Autodesk Inventor part; units mm, degrees
(part 3 of 4)
  line L1957 (8.8556, -3.4816) -> (8.8777, -3.4972)
  line L1958 (8.8777, -3.4972) -> (8.9019, -3.5124)
  line L1959 (8.9019, -3.5124) -> (8.9282, -3.5273)
  line L1960 (8.9282, -3.5273) -> (8.9566, -3.5418)
  line L1961 (8.9566, -3.5418) -> (8.9871, -3.5559)
  line L1962 (9.0196, -3.5695) -> (9.0542, -3.5828)
  line L1963 (11, -4.291) -> (11, -4.7124)
  line L1964 (8.7595, -3.3664) -> (8.7669, -3.3833)
  line L1965 (8.7669, -3.3833) -> (8.7764, -3.4002)
  line L1966 (8.7764, -3.4002) -> (8.788, -3.4169)
  line L1967 (8.788, -3.4169) -> (8.8018, -3.4334)
  line L1968 (8.8176, -3.4497) -> (8.8355, -3.4658)
  line L1969 (8.8355, -3.4658) -> (8.8556, -3.4816)
  line L1970 (8.8018, -3.4334) -> (8.8176, -3.4497)
  line L1971 (11, -10.5741) -> (11, -10.9956)
  line L1972 (9.0542, -9.8659) -> (11, -10.5741)
  line L1973 (9.0196, -9.8527) -> (9.0542, -9.8659)
  line L1974 (8.9871, -9.8391) -> (9.0196, -9.8527)
  line L1975 (8.788, -9.7001) -> (8.8018, -9.7166)
  line L1976 (8.8018, -9.7166) -> (8.8176, -9.7329)
  line L1977 (8.8176, -9.7329) -> (8.8355, -9.749)
  line L1978 (8.8355, -9.749) -> (8.8556, -9.7648)
  line L1979 (8.8556, -9.7648) -> (8.8777, -9.7804)
  line L1980 (8.8777, -9.7804) -> (8.9019, -9.7956)
  line L1981 (8.9019, -9.7956) -> (8.9282, -9.8105)
  line L1982 (8.9282, -9.8105) -> (8.9566, -9.825)
  line L1983 (8.9566, -9.825) -> (8.9871, -9.8391)
  line L1984 (8.7764, -9.6834) -> (8.788, -9.7001)
  line L1985 (8.7669, -9.6665) -> (8.7764, -9.6834)
  line L1986 (8.7595, -9.6495) -> (8.7669, -9.6665)
  line L1987 (8.7542, -9.6325) -> (8.7595, -9.6495)
  line L1988 (8.7511, -9.6154) -> (8.7542, -9.6325)
  line L1989 (8.75, -9.5983) -> (8.7511, -9.6154)
  line L1990 (8.75, -9.4248) -> (8.75, -9.5983)
  line L1991 (8.75, -9.4248) -> (8.75, -9.2513)
  line L1992 (8.75, -9.2513) -> (8.7511, -9.2342)
  line L1993 (8.7511, -9.2342) -> (8.7542, -9.2171)
  line L1994 (8.7542, -9.2171) -> (8.7595, -9.2)
  line L1995 (8.7595, -9.2) -> (8.7669, -9.183)
  line L1996 (8.7669, -9.183) -> (8.7764, -9.1662)
  line L1997 (8.7764, -9.1662) -> (8.788, -9.1495)
  line L1998 (8.8018, -9.133) -> (8.8176, -9.1167)
  line L1999 (8.8176, -9.1167) -> (8.8355, -9.1006)
  line L2000 (8.8355, -9.1006) -> (8.8556, -9.0847)
  line L2001 (8.8556, -9.0847) -> (8.8777, -9.0692)
  line L2002 (8.788, -9.1495) -> (8.8018, -9.133)
  line L2003 (8.8777, -9.0692) -> (8.9019, -9.054)
  line L2004 (8.9019, -9.054) -> (8.9282, -9.0391)
  line L2005 (8.9282, -9.0391) -> (8.9566, -9.0246)
  line L2006 (8.9566, -9.0246) -> (8.9871, -9.0105)
  line L2007 (8.9871, -9.0105) -> (9.0196, -8.9968)
  line L2008 (9.0196, -8.9968) -> (9.0542, -8.9836)
  line L2009 (8.8018, -6.575) -> (8.8176, -6.5913)
  line L2010 (8.8176, -6.5913) -> (8.8355, -6.6074)
  line L2011 (8.8355, -6.6074) -> (8.8556, -6.6232)
  line L2012 (8.8556, -6.6232) -> (8.8777, -6.6388)
  line L2013 (8.8777, -6.6388) -> (8.9019, -6.654)
  line L2014 (8.9019, -6.654) -> (8.9282, -6.6689)
  line L2015 (8.9282, -6.6689) -> (8.9566, -6.6834)
  line L2016 (8.9566, -6.6834) -> (8.9871, -6.6975)
  line L2017 (8.9871, -6.6975) -> (9.0196, -6.7111)
  line L2018 (8.75, 0) -> (8.75, -0.1735)
  line L2019 (8.75, -0.1735) -> (8.7511, -0.1906)
  line L2020 (8.7511, -0.1906) -> (8.7542, -0.2077)
  line L2021 (8.7542, -0.2077) -> (8.7595, -0.2248)
  line L2022 (8.7595, -0.2248) -> (8.7669, -0.2417)
  line L2023 (8.7669, -0.2417) -> (8.7764, -0.2586)
  line L2024 (8.7764, -0.2586) -> (8.788, -0.2753)
  line L2025 (8.788, -0.2753) -> (8.8018, -0.2918)
  line L2026 (9.0542, -0.4412) -> (11, -1.1494)
  line L2027 (11, -1.1494) -> (11, -1.5708)
  line L2028 (8.9566, -2.7414) -> (8.9871, -2.7273)
  line L2029 (8.9871, -2.7273) -> (9.0196, -2.7136)
  line L2030 (9.0196, -2.7136) -> (9.0542, -2.7004)
  line L2031 (11, -1.9922) -> (11, -1.5708)
  line L2032 (9.0542, -2.7004) -> (11, -1.9922)
  line L2033 (9.0542, -8.9836) -> (11, -8.2754)
  line L2034 (9.0196, -6.7111) -> (9.0542, -6.7243)
  line L2035 (9.0542, -6.7243) -> (11, -7.4326)
  line L2036 (11, -8.2754) -> (11, -7.854)
  line L2037 (11, -7.4326) -> (11, -7.854)
  line L2038 (8.7511, -34.7481) -> (8.7542, -34.7652)
  line L2039 (8.8018, -34.8493) -> (8.8176, -34.8656)
  line L2040 (8.788, -34.8328) -> (8.8018, -34.8493)
  line L2041 (8.7764, -34.8161) -> (8.788, -34.8328)
  line L2042 (8.7669, -34.7992) -> (8.7764, -34.8161)
  line L2043 (8.7595, -34.7823) -> (8.7669, -34.7992)
  line L2044 (8.75, -34.731) -> (8.7511, -34.7481)
  line L2045 (8.75, -34.5575) -> (8.75, -34.731)
  line L2046 (8.7542, -34.7652) -> (8.7595, -34.7823)
  line L2047 (8.75, -34.5575) -> (8.75, -34.384)
  line L2048 (8.75, -34.384) -> (8.7511, -34.3669)
  line L2049 (8.8556, -34.2175) -> (8.8777, -34.2019)
  line L2050 (8.8355, -34.2333) -> (8.8556, -34.2175)
  line L2051 (8.8176, -34.2494) -> (8.8355, -34.2333)
  line L2052 (8.8018, -34.2657) -> (8.8176, -34.2494)
  line L2053 (8.788, -34.2822) -> (8.8018, -34.2657)
  line L2054 (8.7764, -34.2989) -> (8.788, -34.2822)
  line L2055 (8.7669, -34.3158) -> (8.7764, -34.2989)
  line L2056 (8.7595, -34.3327) -> (8.7669, -34.3158)
  line L2057 (8.7542, -34.3498) -> (8.7595, -34.3327)
  line L2058 (8.7511, -34.3669) -> (8.7542, -34.3498)
  line L2059 (9.0542, -34.1164) -> (11, -33.4082)
  line L2060 (8.8777, -31.7715) -> (8.9019, -31.7867)
  line L2061 (8.9019, -31.7867) -> (8.9282, -31.8016)
  line L2062 (8.9282, -31.8016) -> (8.9566, -31.8161)
  line L2063 (8.9566, -31.8161) -> (8.9871, -31.8302)
  line L2064 (8.9871, -31.8302) -> (9.0196, -31.8439)
  line L2065 (9.0196, -31.8439) -> (9.0542, -31.8571)
  line L2066 (9.0542, -31.8571) -> (11, -32.5653)
  line L2067 (11, -33.4082) -> (11, -32.9867)
  line L2068 (11, -32.5653) -> (11, -32.9867)
  line L2069 (8.8176, -34.8656) -> (8.8355, -34.8817)
  line L2070 (8.8355, -34.8817) -> (8.8556, -34.8976)
  line L2071 (8.8556, -34.8976) -> (8.8777, -34.9131)
  line L2072 (8.8777, -34.9131) -> (8.9019, -34.9283)
  line L2073 (8.9019, -34.9283) -> (8.9282, -34.9432)
  line L2074 (8.9282, -34.9432) -> (8.9566, -34.9577)
  line L2075 (8.9566, -34.9577) -> (8.9871, -34.9718)
  line L2076 (8.9871, -34.9718) -> (9.0196, -34.9855)
  line L2077 (9.0196, -34.9855) -> (9.0542, -34.9987)
  line L2078 (8.8777, -34.2019) -> (8.9019, -34.1867)
  line L2079 (8.9019, -34.1867) -> (8.9282, -34.1718)
  line L2080 (8.9282, -34.1718) -> (8.9566, -34.1573)
  line L2081 (8.9566, -34.1573) -> (8.9871, -34.1432)
  line L2082 (9.0196, -34.1296) -> (9.0542, -34.1164)
  line L2083 (8.9871, -34.1432) -> (9.0196, -34.1296)
  line L2084 (8.9282, -28.66) -> (8.9566, -28.6745)
  line L2085 (8.9566, -28.6745) -> (8.9871, -28.6886)
  line L2086 (8.9871, -28.6886) -> (9.0196, -28.7023)
  line L2087 (9.0542, -28.7155) -> (11, -29.4237)
  line L2088 (8.9282, -31.0302) -> (8.9566, -31.0157)
  line L2089 (8.9566, -31.0157) -> (8.9871, -31.0016)
  line L2090 (8.9871, -31.0016) -> (9.0196, -30.988)
  line L2091 (9.0542, -30.9748) -> (11, -30.2666)
  line L2092 (11, -30.2666) -> (11, -29.8451)
  line L2093 (11, -29.4237) -> (11, -29.8451)
  line L2094 (9.0196, -28.7023) -> (9.0542, -28.7155)
  line L2095 (9.0196, -30.988) -> (9.0542, -30.9748)
  line L2096 (8.75, -6.2832) -> (7.8414, -6.2832)
  line L2097 (8.75, -6.2832) -> (8.75, -6.4567)
  line L2098 (8.75, -6.4567) -> (8.7511, -6.4738)
  line L2099 (8.7511, -6.4738) -> (8.7542, -6.4909)
  line L2100 (8.7542, -6.4909) -> (8.7595, -6.508)
  line L2101 (8.7595, -6.508) -> (8.7669, -6.5249)
  line L2102 (8.7669, -6.5249) -> (8.7764, -6.5418)
  line L2103 (8.7764, -6.5418) -> (8.788, -6.5585)
  line L2104 (8.788, -6.5585) -> (8.8018, -6.575)
  line L2105 (9.0542, -34.9987) -> (11, -35.7069)
  line L2106 (11, -35.7069) -> (11, -36.1283)
  line L2107 (11, -36.5497) -> (11, -36.1283)
  line L2108 (9.0542, -37.258) -> (11, -36.5497)
  line L2109 (9.0196, -37.2712) -> (9.0542, -37.258)
  line L2110 (8.9871, -37.2848) -> (9.0196, -37.2712)
  line L2111 (8.9566, -37.2989) -> (8.9871, -37.2848)
  line L2112 (8.9282, -37.3134) -> (8.9566, -37.2989)
  line L2113 (8.9019, -37.3283) -> (8.9282, -37.3134)
  line L2114 (8.8777, -37.3435) -> (8.9019, -37.3283)
  line L2115 (8.8556, -37.3591) -> (8.8777, -37.3435)
  line L2116 (8.788, -75.123) -> (8.8018, -75.1064)
  line L2117 (8.7764, -75.1397) -> (8.788, -75.123)
  line L2118 (8.7669, -75.1565) -> (8.7764, -75.1397)
  line L2119 (8.7595, -75.1735) -> (8.7669, -75.1565)
  line L2120 (8.7542, -75.1905) -> (8.7595, -75.1735)
  line L2121 (8.7511, -75.2076) -> (8.7542, -75.1905)
  line L2122 (8.75, -75.2247) -> (8.7511, -75.2076)
  line L2123 (8.75, -75.3982) -> (8.75, -75.2247)
  line L2124 (9.0196, -72.6846) -> (9.0542, -72.6978)
  line L2125 (8.9871, -72.6709) -> (9.0196, -72.6846)
  line L2126 (8.9566, -72.6568) -> (8.9871, -72.6709)
  line L2127 (8.9282, -72.6423) -> (8.9566, -72.6568)
  line L2128 (8.9019, -72.6274) -> (8.9282, -72.6423)
  line L2129 (8.8777, -72.6122) -> (8.9019, -72.6274)
  line L2130 (8.8556, -72.5967) -> (8.8777, -72.6122)
  line L2131 (8.8355, -72.5808) -> (8.8556, -72.5967)
  line L2132 (8.8176, -72.5648) -> (8.8355, -72.5808)
  line L2133 (8.8018, -72.5484) -> (8.8176, -72.5648)
  line L2134 (8.788, -72.5319) -> (8.8018, -72.5484)
  line L2135 (8.7764, -72.5152) -> (8.788, -72.5319)
  line L2136 (8.8176, -75.0901) -> (8.8355, -75.074)
  line L2137 (8.8018, -75.1064) -> (8.8176, -75.0901)
  line L2138 (8.8355, -75.074) -> (8.8556, -75.0582)
  line L2139 (8.8556, -75.0582) -> (8.8777, -75.0426)
  line L2140 (8.8777, -75.0426) -> (8.9019, -75.0274)
  line L2141 (8.9019, -75.0274) -> (8.9282, -75.0125)
  line L2142 (8.9282, -75.0125) -> (8.9566, -74.998)
  line L2143 (8.9566, -74.998) -> (8.9871, -74.9839)
  line L2144 (8.9871, -74.9839) -> (9.0196, -74.9703)
  line L2145 (8.7669, -72.4984) -> (8.7764, -72.5152)
  line L2146 (8.7595, -72.4814) -> (8.7669, -72.4984)
  line L2147 (8.7542, -72.4644) -> (8.7595, -72.4814)
  line L2148 (8.7511, -72.4472) -> (8.7542, -72.4644)
  line L2149 (8.75, -72.4301) -> (8.7511, -72.4472)
  line L2150 (8.75, -72.2566) -> (8.75, -72.4301)
  line L2151 (8.75, -72.2566) -> (8.75, -72.0831)
  line L2152 (8.75, -72.0831) -> (8.7511, -72.066)
  line L2153 (8.7511, -72.066) -> (8.7542, -72.0489)
  line L2154 (8.7542, -72.0489) -> (8.7595, -72.0319)
  line L2155 (8.7595, -72.0319) -> (8.7669, -72.0149)
  line L2156 (8.7669, -72.0149) -> (8.7764, -71.9981)
  line L2157 (8.7595, -69.3398) -> (8.7669, -69.3568)
  line L2158 (8.7542, -69.3228) -> (8.7595, -69.3398)
  line L2159 (8.7511, -69.3057) -> (8.7542, -69.3228)
  line L2160 (8.75, -69.2885) -> (8.7511, -69.3057)
  line L2161 (8.75, -69.115) -> (8.75, -69.2885)
  line L2162 (8.7764, -71.9981) -> (8.788, -71.9814)
  line L2163 (8.788, -71.9814) -> (8.8018, -71.9648)
  line L2164 (8.8018, -71.9648) -> (8.8176, -71.9485)
  line L2165 (8.8176, -71.9485) -> (8.8355, -71.9324)
  line L2166 (8.8355, -71.9324) -> (8.8556, -71.9166)
  line L2167 (8.8556, -71.9166) -> (8.8777, -71.901)
  line L2168 (8.8777, -71.901) -> (8.9019, -71.8858)
  line L2169 (8.9019, -71.8858) -> (8.9282, -71.8709)
  line L2170 (8.7669, -69.3568) -> (8.7764, -69.3736)
  line L2171 (8.9871, -71.8423) -> (9.0196, -71.8287)
  line L2172 (8.9566, -71.8564) -> (8.9871, -71.8423)
  line L2173 (8.9282, -71.8709) -> (8.9566, -71.8564)
  line L2174 (9.0542, -69.5562) -> (11, -70.2644)
  line L2175 (9.0196, -71.8287) -> (9.0542, -71.8155)
  line L2176 (9.0542, -71.8155) -> (11, -71.1073)
  line L2177 (11, -70.2644) -> (11, -70.6858)
  line L2178 (11, -71.1073) -> (11, -70.6858)
  line L2179 (8.7764, -68.8565) -> (8.788, -68.8398)
  line L2180 (8.788, -68.8398) -> (8.8018, -68.8232)
  line L2181 (8.8018, -68.8232) -> (8.8176, -68.8069)
  line L2182 (8.8176, -68.8069) -> (8.8355, -68.7908)
  line L2183 (8.8355, -68.7908) -> (8.8556, -68.775)
  line L2184 (8.8556, -68.775) -> (8.8777, -68.7595)
  line L2185 (9.0196, -68.6871) -> (9.0542, -68.6739)
  line L2186 (8.9871, -68.7008) -> (9.0196, -68.6871)
  line L2187 (8.9566, -68.7149) -> (8.9871, -68.7008)
  line L2188 (8.9282, -68.7294) -> (8.9566, -68.7149)
  line L2189 (8.8777, -68.7595) -> (8.9019, -68.7442)
  line L2190 (8.9019, -68.7442) -> (8.9282, -68.7294)
  line L2191 (9.0542, -68.6739) -> (11, -67.9657)
  line L2192 (11, -67.9657) -> (11, -67.5442)
  line L2193 (11, -67.1228) -> (11, -67.5442)
  line L2194 (9.0542, -66.4146) -> (11, -67.1228)
  line L2195 (9.0196, -66.4014) -> (9.0542, -66.4146)
  line L2196 (8.9871, -66.3877) -> (9.0196, -66.4014)
  line L2197 (8.9566, -66.3736) -> (8.9871, -66.3877)
  line L2198 (8.9282, -66.3591) -> (8.9566, -66.3736)
  line L2199 (8.9019, -66.3443) -> (8.9282, -66.3591)
  line L2200 (8.8777, -66.329) -> (8.9019, -66.3443)
  line L2201 (8.8556, -66.3135) -> (8.8777, -66.329)
  line L2202 (8.8355, -66.2977) -> (8.8556, -66.3135)
  line L2203 (8.8176, -66.2816) -> (8.8355, -66.2977)
  line L2204 (8.8018, -66.2652) -> (8.8176, -66.2816)
  line L2205 (8.788, -66.2487) -> (8.8018, -66.2652)
  line L2206 (8.7764, -66.232) -> (8.788, -66.2487)
  line L2207 (8.7669, -66.2152) -> (8.7764, -66.232)
  line L2208 (8.7595, -66.1982) -> (8.7669, -66.2152)
  line L2209 (8.7511, -66.1641) -> (8.7542, -66.1812)
  line L2210 (8.7542, -66.1812) -> (8.7595, -66.1982)
  line L2211 (8.75, -65.9734) -> (8.75, -65.8)
  line L2212 (8.75, -65.8) -> (8.7511, -65.7828)
  line L2213 (8.7511, -65.7828) -> (8.7542, -65.7657)
  line L2214 (8.7542, -65.7657) -> (8.7595, -65.7487)
  line L2215 (8.7595, -65.7487) -> (8.7669, -65.7317)
  line L2216 (8.7669, -65.7317) -> (8.7764, -65.7149)
  line L2217 (8.7764, -65.7149) -> (8.788, -65.6982)
  line L2218 (8.788, -65.6982) -> (8.8018, -65.6816)
  line L2219 (8.8018, -65.6816) -> (8.8176, -65.6653)
  line L2220 (8.8176, -65.6653) -> (8.8355, -65.6492)
  line L2221 (8.8355, -65.6492) -> (8.8556, -65.6334)
  line L2222 (8.8556, -65.6334) -> (8.8777, -65.6179)
  line L2223 (8.8777, -65.6179) -> (8.9019, -65.6026)
  line L2224 (8.9019, -65.6026) -> (8.9282, -65.5878)
  line L2225 (8.9566, -65.5733) -> (8.9871, -65.5592)
  line L2226 (8.9871, -65.5592) -> (9.0196, -65.5455)
  line L2227 (9.0196, -65.5455) -> (9.0542, -65.5323)
  line L2228 (8.9282, -65.5878) -> (8.9566, -65.5733)
  line L2229 (11, -64.8241) -> (11, -64.4026)
  line L2230 (9.0542, -63.273) -> (11, -63.9812)
  line L2231 (9.0542, -65.5323) -> (11, -64.8241)
  line L2232 (11, -63.9812) -> (11, -64.4026)
  line L2233 (9.0196, -69.543) -> (9.0542, -69.5562)
  line L2234 (8.9871, -69.5293) -> (9.0196, -69.543)
  line L2235 (8.9566, -69.5152) -> (8.9871, -69.5293)
  line L2236 (8.9282, -69.5007) -> (8.9566, -69.5152)
  line L2237 (8.9019, -69.4858) -> (8.9282, -69.5007)
  line L2238 (8.8556, -69.4551) -> (8.8777, -69.4706)
  line L2239 (8.8355, -69.4392) -> (8.8556, -69.4551)
  line L2240 (8.8176, -69.4232) -> (8.8355, -69.4392)
  line L2241 (8.8018, -69.4068) -> (8.8176, -69.4232)
  line L2242 (8.788, -69.3903) -> (8.8018, -69.4068)
  line L2243 (8.7764, -69.3736) -> (8.788, -69.3903)
  line L2244 (8.8777, -69.4706) -> (8.9019, -69.4858)
  line L2245 (9.0542, -72.6978) -> (11, -73.406)
  line L2246 (11, -73.406) -> (11, -73.8274)
  line L2247 (11, -74.2489) -> (11, -73.8274)
  line L2248 (9.0542, -74.9571) -> (11, -74.2489)
  line L2249 (9.0196, -74.9703) -> (9.0542, -74.9571)
  line L2250 (8.75, -75.3982) -> (8.75, -75.5717)
  line L2251 (8.75, -75.5717) -> (8.7511, -75.5888)
  line L2252 (8.7511, -75.5888) -> (8.7542, -75.6059)
  line L2253 (8.7542, -75.6059) -> (8.7595, -75.623)
  line L2254 (8.7595, -75.623) -> (8.7669, -75.64)
  line L2255 (8.7669, -75.64) -> (8.7764, -75.6568)
  line L2256 (8.7764, -75.6568) -> (8.788, -75.6735)
  line L2257 (8.788, -75.6735) -> (8.8018, -75.69)
  line L2258 (8.8176, -75.7063) -> (8.8355, -75.7224)
  line L2259 (8.8018, -75.69) -> (8.8176, -75.7063)
  line L2260 (8.8355, -75.7224) -> (8.8556, -75.7383)
  line L2261 (8.8777, -75.7538) -> (8.9019, -75.769)
  line L2262 (8.9019, -75.769) -> (8.9282, -75.7839)
  line L2263 (8.9282, -75.7839) -> (8.9566, -75.7984)
  line L2264 (8.9566, -75.7984) -> (8.9871, -75.8125)
  line L2265 (8.8556, -75.7383) -> (8.8777, -75.7538)
  line L2266 (9.0196, -63.2598) -> (9.0542, -63.273)
  line L2267 (8.9871, -63.2461) -> (9.0196, -63.2598)
  line L2268 (8.9566, -63.232) -> (8.9871, -63.2461)
  line L2269 (8.9282, -63.2175) -> (8.9566, -63.232)
  line L2270 (8.9019, -63.2027) -> (8.9282, -63.2175)
  line L2271 (8.8777, -63.1874) -> (8.9019, -63.2027)
  line L2272 (8.8556, -63.1719) -> (8.8777, -63.1874)
  line L2273 (8.8355, -63.1561) -> (8.8556, -63.1719)
  line L2274 (8.7669, -63.0736) -> (8.7764, -63.0904)
  line L2275 (8.7595, -63.0566) -> (8.7669, -63.0736)
  line L2276 (8.7542, -63.0396) -> (8.7595, -63.0566)
  line L2277 (8.7511, -63.0225) -> (8.7542, -63.0396)
  line L2278 (8.75, -63.0053) -> (8.7511, -63.0225)
  line L2279 (8.75, -62.8319) -> (8.75, -63.0053)
  line L2280 (9.0196, -88.3925) -> (9.0542, -88.4058)
  line L2281 (9.0542, -88.4058) -> (11, -89.114)
  line L2282 (8.9566, -90.706) -> (8.9871, -90.6919)
  line L2283 (8.9871, -90.6919) -> (9.0196, -90.6782)
  line L2284 (9.0196, -90.6782) -> (9.0542, -90.665)
  line L2285 (9.0542, -90.665) -> (11, -89.9568)
  line L2286 (11, -89.9568) -> (11, -89.5354)
  line L2287 (11, -89.114) -> (11, -89.5354)
  line L2288 (8.9282, -90.7205) -> (8.9566, -90.706)
  line L2289 (8.7669, -90.8645) -> (8.7764, -90.8476)
  line L2290 (8.9019, -90.7354) -> (8.9282, -90.7205)
  line L2291 (8.8777, -90.7506) -> (8.9019, -90.7354)
  line L2292 (8.8556, -90.7661) -> (8.8777, -90.7506)
  line L2293 (8.8355, -90.782) -> (8.8556, -90.7661)
  line L2294 (8.8176, -90.7981) -> (8.8355, -90.782)
  line L2295 (8.8018, -90.8144) -> (8.8176, -90.7981)
  line L2296 (8.788, -90.8309) -> (8.8018, -90.8144)
  line L2297 (8.75, -91.1062) -> (8.75, -90.9327)
  line L2298 (8.75, -91.1062) -> (8.75, -91.2797)
  line L2299 (8.7764, -90.8476) -> (8.788, -90.8309)
  line L2300 (8.75, -91.2797) -> (8.7511, -91.2968)
  line L2301 (8.7511, -91.2968) -> (8.7542, -91.3139)
  line L2302 (8.7542, -91.3139) -> (8.7595, -91.331)
  line L2303 (8.7595, -91.331) -> (8.7669, -91.3479)
  line L2304 (8.7669, -91.3479) -> (8.7764, -91.3648)
  line L2305 (8.7764, -91.3648) -> (8.788, -91.3815)
  line L2306 (8.788, -91.3815) -> (8.8018, -91.398)
  line L2307 (8.8018, -91.398) -> (8.8176, -91.4143)
  line L2308 (8.8176, -91.4143) -> (8.8355, -91.4304)
  line L2309 (8.8355, -91.4304) -> (8.8556, -91.4462)
  line L2310 (8.8556, -91.4462) -> (8.8777, -91.4618)
  line L2311 (8.8777, -91.4618) -> (8.9019, -91.477)
  line L2312 (8.9019, -91.477) -> (8.9282, -91.4919)
  line L2313 (8.9282, -91.4919) -> (8.9566, -91.5064)
  line L2314 (8.9566, -91.5064) -> (8.9871, -91.5205)
  line L2315 (8.9871, -91.5205) -> (9.0196, -91.5341)
  line L2316 (9.0196, -91.5341) -> (9.0542, -91.5473)
  line L2317 (8.9871, -93.8335) -> (9.0196, -93.8198)
  line L2318 (9.0196, -93.8198) -> (9.0542, -93.8066)
  line L2319 (9.0542, -93.8066) -> (11, -93.0984)
  line L2320 (11, -93.0984) -> (11, -92.677)
  line L2321 (11, -92.2556) -> (11, -92.677)
  line L2322 (9.0542, -91.5473) -> (11, -92.2556)
  line L2323 (8.9566, -93.8476) -> (8.9871, -93.8335)
  line L2324 (8.75, -90.9327) -> (8.7511, -90.9156)
  line L2325 (8.7669, -94.0061) -> (8.7764, -93.9892)
  line L2326 (8.7511, -94.0572) -> (8.7542, -94.0401)
  line L2327 (8.75, -94.0743) -> (8.7511, -94.0572)
  line L2328 (8.75, -94.2478) -> (7.8414, -94.2478)
  line L2329 (8.75, -94.2478) -> (8.75, -94.0743)
  line L2330 (8.7595, -94.023) -> (8.7669, -94.0061)
  line L2331 (8.9282, -93.8621) -> (8.9566, -93.8476)
  line L2332 (8.9019, -93.877) -> (8.9282, -93.8621)
  line L2333 (8.8777, -93.8922) -> (8.9019, -93.877)
  line L2334 (8.8556, -93.9077) -> (8.8777, -93.8922)
  line L2335 (8.8355, -93.9236) -> (8.8556, -93.9077)
  line L2336 (8.8176, -93.9397) -> (8.8355, -93.9236)
  line L2337 (8.8018, -93.956) -> (8.8176, -93.9397)
  line L2338 (8.788, -93.9725) -> (8.8018, -93.956)
  line L2339 (8.7764, -93.9892) -> (8.788, -93.9725)
  line L2340 (8.7542, -94.0401) -> (8.7595, -94.023)
  line L2341 (8.75, -94.2478) -> (8.75, -94.4213)
  line L2342 (8.75, -94.4213) -> (8.7511, -94.4384)
  line L2343 (8.7511, -94.4384) -> (8.7542, -94.4555)
  line L2344 (8.7595, -94.4725) -> (8.7669, -94.4895)
  line L2345 (8.7669, -94.4895) -> (8.7764, -94.5064)
  line L2346 (8.7542, -94.4555) -> (8.7595, -94.4725)
  line L2347 (8.9282, -97.0037) -> (8.9566, -96.9892)
  line L2348 (8.9019, -97.0186) -> (8.9282, -97.0037)
  line L2349 (8.8777, -97.0338) -> (8.9019, -97.0186)
  line L2350 (8.8556, -97.0493) -> (8.8777, -97.0338)
  line L2351 (8.8176, -97.0813) -> (8.8355, -97.0652)
  line L2352 (8.8018, -97.0976) -> (8.8176, -97.0813)
  line L2353 (8.788, -97.1141) -> (8.8018, -97.0976)
  line L2354 (8.7764, -97.1308) -> (8.788, -97.1141)
  line L2355 (8.7595, -97.1646) -> (8.7669, -97.1476)
  line L2356 (8.7542, -97.1816) -> (8.7595, -97.1646)
  line L2357 (8.7511, -97.1988) -> (8.7542, -97.1816)
  line L2358 (8.8355, -97.0652) -> (8.8556, -97.0493)
  line L2359 (8.75, -97.3894) -> (8.75, -97.2159)
  line L2360 (8.75, -97.3894) -> (8.75, -97.5629)
  line L2361 (8.75, -97.5629) -> (8.7511, -97.58)
  line L2362 (8.7511, -97.58) -> (8.7542, -97.5971)
  line L2363 (8.7542, -97.5971) -> (8.7595, -97.6141)
  line L2364 (8.7595, -97.6141) -> (8.7669, -97.6311)
  line L2365 (8.75, -97.2159) -> (8.7511, -97.1988)
  line L2366 (8.8777, -94.6034) -> (8.9019, -94.6186)
  line L2367 (8.9019, -94.6186) -> (8.9282, -94.6335)
  line L2368 (8.9282, -94.6335) -> (8.9566, -94.648)
  line L2369 (8.8556, -94.5878) -> (8.8777, -94.6034)
  line L2370 (8.7764, -94.5064) -> (8.788, -94.5231)
  line L2371 (8.788, -94.5231) -> (8.8018, -94.5396)
  line L2372 (8.8018, -94.5396) -> (8.8176, -94.5559)
  line L2373 (8.8176, -94.5559) -> (8.8355, -94.572)
  line L2374 (8.8355, -94.572) -> (8.8556, -94.5878)
  line L2375 (8.7669, -97.1476) -> (8.7764, -97.1308)
  line L2376 (8.7669, -97.6311) -> (8.7764, -97.6479)
  line L2377 (8.788, -97.6646) -> (8.8018, -97.6812)
  line L2378 (8.8018, -97.6812) -> (8.8176, -97.6975)
  line L2379 (8.8176, -97.6975) -> (8.8355, -97.7136)
  line L2380 (8.8355, -97.7136) -> (8.8556, -97.7294)
  line L2381 (8.8556, -97.7294) -> (8.8777, -97.745)
  line L2382 (8.7764, -97.6479) -> (8.788, -97.6646)
  line L2383 (8.8777, -97.745) -> (8.9019, -97.7602)
  line L2384 (8.9019, -97.7602) -> (8.9282, -97.7751)
  line L2385 (8.9566, -97.7896) -> (8.9871, -97.8037)
  line L2386 (8.9871, -97.8037) -> (9.0196, -97.8173)
  line L2387 (9.0196, -97.8173) -> (9.0542, -97.8305)
  line L2388 (9.0542, -97.8305) -> (11, -98.5387)
  line L2389 (11, -98.5387) -> (11, -98.9602)
  line L2390 (8.9282, -97.7751) -> (8.9566, -97.7896)
  line L2391 (8.9566, -94.648) -> (8.9871, -94.6621)
  line L2392 (8.9871, -94.6621) -> (9.0196, -94.6757)
  line L2393 (9.0196, -94.6757) -> (9.0542, -94.6889)
  line L2394 (9.0542, -94.6889) -> (11, -95.3971)
  line L2395 (11, -95.3971) -> (11, -95.8186)
  line L2396 (8.9871, -96.9751) -> (9.0196, -96.9614)
  line L2397 (9.0196, -96.9614) -> (9.0542, -96.9482)
  line L2398 (9.0542, -96.9482) -> (11, -96.24)
  line L2399 (11, -96.24) -> (11, -95.8186)
  line L2400 (8.9566, -96.9892) -> (8.9871, -96.9751)
  line L2401 (9.0542, -85.2642) -> (11, -85.9724)
  line L2402 (9.0542, -87.5234) -> (11, -86.8152)
  line L2403 (11, -85.9724) -> (11, -86.3938)
  line L2404 (11, -86.8152) -> (11, -86.3938)
  line L2405 (8.9871, -85.2373) -> (9.0196, -85.251)
  line L2406 (8.9871, -75.8125) -> (9.0196, -75.8262)
  line L2407 (9.0196, -75.8262) -> (9.0542, -75.8394)
  line L2408 (9.0542, -75.8394) -> (11, -76.5476)
  line L2409 (11, -76.5476) -> (11, -76.969)
  line L2410 (11, -77.3904) -> (11, -76.969)
  line L2411 (9.0542, -78.0987) -> (11, -77.3904)
  line L2412 (9.0196, -78.1119) -> (9.0542, -78.0987)
  line L2413 (8.8018, -78.248) -> (8.8176, -78.2317)
  line L2414 (8.8176, -78.2317) -> (8.8355, -78.2156)
  line L2415 (8.8355, -78.2156) -> (8.8556, -78.1998)
  line L2416 (8.8556, -78.1998) -> (8.8777, -78.1842)
  line L2417 (8.8777, -78.1842) -> (8.9019, -78.169)
  line L2418 (8.9019, -78.169) -> (8.9282, -78.1541)
  line L2419 (8.9282, -78.1541) -> (8.9566, -78.1396)
  line L2420 (8.9566, -78.1396) -> (8.9871, -78.1255)
  line L2421 (8.9871, -78.1255) -> (9.0196, -78.1119)
  line L2422 (8.7511, -78.3492) -> (8.7542, -78.3321)
  line L2423 (8.788, -78.8151) -> (8.8018, -78.8316)
  line L2424 (8.7764, -78.7984) -> (8.788, -78.8151)
  line L2425 (8.7669, -78.7815) -> (8.7764, -78.7984)
  line L2426 (8.7595, -78.7646) -> (8.7669, -78.7815)
  line L2427 (8.7542, -78.7475) -> (8.7595, -78.7646)
  line L2428 (8.7511, -78.7304) -> (8.7542, -78.7475)
  line L2429 (8.75, -78.5398) -> (8.75, -78.7133)
  line L2430 (8.75, -78.5398) -> (8.75, -78.3663)
  line L2431 (8.75, -78.3663) -> (8.7511, -78.3492)
  line L2432 (8.7542, -78.3321) -> (8.7595, -78.315)
  line L2433 (8.7595, -78.315) -> (8.7669, -78.2981)
  line L2434 (8.7669, -78.2981) -> (8.7764, -78.2812)
  line L2435 (8.7764, -78.2812) -> (8.788, -78.2645)
  line L2436 (8.788, -78.2645) -> (8.8018, -78.248)
  line L2437 (8.75, -78.7133) -> (8.7511, -78.7304)
  line L2438 (9.0196, -78.9678) -> (9.0542, -78.981)
  line L2439 (8.9871, -78.9541) -> (9.0196, -78.9678)
  line L2440 (8.9566, -78.94) -> (8.9871, -78.9541)
  line L2441 (8.9282, -78.9255) -> (8.9566, -78.94)
  line L2442 (8.9019, -78.9106) -> (8.9282, -78.9255)
  line L2443 (8.8777, -78.8954) -> (8.9019, -78.9106)
  line L2444 (8.8556, -78.8799) -> (8.8777, -78.8954)
  line L2445 (8.8355, -78.864) -> (8.8556, -78.8799)
  line L2446 (8.8176, -78.8479) -> (8.8355, -78.864)
  line L2447 (8.8018, -78.8316) -> (8.8176, -78.8479)
  line L2448 (9.0196, -81.2535) -> (9.0542, -81.2402)
  line L2449 (9.0542, -78.981) -> (11, -79.6892)
  line L2450 (8.9282, -81.2957) -> (8.9566, -81.2812)
  line L2451 (8.9566, -81.2812) -> (8.9871, -81.2671)
  line L2452 (8.9871, -81.2671) -> (9.0196, -81.2535)
  line L2453 (9.0542, -81.2402) -> (11, -80.532)
  line L2454 (11, -79.6892) -> (11, -80.1106)
  line L2455 (11, -80.532) -> (11, -80.1106)
  line L2456 (8.7542, -81.8891) -> (8.7595, -81.9062)
  line L2457 (8.7511, -81.872) -> (8.7542, -81.8891)
  line L2458 (8.75, -81.8549) -> (8.7511, -81.872)
  line L2459 (8.75, -81.6814) -> (8.75, -81.8549)
  line L2460 (8.75, -81.6814) -> (8.75, -81.5079)
  line L2461 (8.75, -81.5079) -> (8.7511, -81.4908)
  line L2462 (8.7511, -81.4908) -> (8.7542, -81.4737)
  line L2463 (8.7542, -81.4737) -> (8.7595, -81.4566)
  line L2464 (9.0542, -84.3818) -> (11, -83.6736)
  line L2465 (9.0542, -82.1226) -> (11, -82.8308)
  line L2466 (11, -82.8308) -> (11, -83.2522)
  line L2467 (11, -83.6736) -> (11, -83.2522)
  line L2468 (8.7595, -84.5982) -> (8.7669, -84.5813)
  line L2469 (8.7669, -84.5813) -> (8.7764, -84.5644)
  line L2470 (8.7764, -84.5644) -> (8.788, -84.5477)
  line L2471 (8.788, -84.5477) -> (8.8018, -84.5312)
  line L2472 (8.8018, -84.5312) -> (8.8176, -84.5149)
  line L2473 (8.8176, -84.5149) -> (8.8355, -84.4988)
  line L2474 (8.8355, -84.4988) -> (8.8556, -84.483)
  line L2475 (8.8556, -84.483) -> (8.8777, -84.4674)
  line L2476 (8.8777, -84.4674) -> (8.9019, -84.4522)
  line L2477 (8.9019, -84.4522) -> (8.9282, -84.4373)
  line L2478 (8.9282, -84.4373) -> (8.9566, -84.4228)
  line L2479 (8.9566, -84.4228) -> (8.9871, -84.4087)
  line L2480 (8.9871, -84.4087) -> (9.0196, -84.395)
  line L2481 (9.0196, -84.395) -> (9.0542, -84.3818)
  line L2482 (8.7542, -84.6153) -> (8.7595, -84.5982)
  line L2483 (8.7511, -84.6324) -> (8.7542, -84.6153)
  line L2484 (8.75, -84.6495) -> (8.7511, -84.6324)
  line L2485 (8.75, -84.823) -> (8.75, -84.6495)
  line L2486 (8.75, -84.823) -> (8.75, -84.9965)
  line L2487 (8.75, -84.9965) -> (8.7511, -85.0136)
  line L2488 (8.7511, -85.0136) -> (8.7542, -85.0307)
  line L2489 (8.7542, -85.0307) -> (8.7595, -85.0478)
  line L2490 (8.8018, -85.1148) -> (8.8176, -85.1311)
  line L2491 (8.788, -85.0983) -> (8.8018, -85.1148)
  line L2492 (8.7669, -85.0647) -> (8.7764, -85.0816)
  line L2493 (8.7764, -85.0816) -> (8.788, -85.0983)
  line L2494 (8.8176, -85.1311) -> (8.8355, -85.1472)
  line L2495 (8.7595, -85.0478) -> (8.7669, -85.0647)
  line L2496 (8.9019, -85.1938) -> (8.9282, -85.2087)
  line L2497 (8.9282, -85.2087) -> (8.9566, -85.2232)
  line L2498 (8.7669, -87.7229) -> (8.7764, -87.706)
  line L2499 (8.9566, -87.5644) -> (8.9871, -87.5503)
  line L2500 (8.9871, -87.5503) -> (9.0196, -87.5366)
  line L2501 (9.0196, -87.5366) -> (9.0542, -87.5234)
  line L2502 (8.9282, -87.5789) -> (8.9566, -87.5644)
  line L2503 (8.9019, -87.5938) -> (8.9282, -87.5789)
  line L2504 (8.8777, -87.609) -> (8.9019, -87.5938)
  line L2505 (8.8355, -87.6404) -> (8.8556, -87.6246)
  line L2506 (8.8176, -87.6565) -> (8.8355, -87.6404)
  line L2507 (8.8018, -87.6728) -> (8.8176, -87.6565)
  line L2508 (8.788, -87.6893) -> (8.8018, -87.6728)
  line L2509 (8.7764, -87.706) -> (8.788, -87.6893)
  line L2510 (8.8556, -87.6246) -> (8.8777, -87.609)
  line L2511 (8.75, -87.7911) -> (8.7511, -87.774)
  line L2512 (8.7511, -87.774) -> (8.7542, -87.7569)
  line L2513 (8.7542, -87.7569) -> (8.7595, -87.7398)
  line L2514 (8.7595, -87.7398) -> (8.7669, -87.7229)
  line L2515 (8.75, -87.9646) -> (8.75, -87.7911)
  line L2516 (8.788, -88.2399) -> (8.8018, -88.2564)
  line L2517 (8.7764, -88.2232) -> (8.788, -88.2399)
  line L2518 (8.7595, -88.1894) -> (8.7669, -88.2063)
  line L2519 (8.7542, -88.1723) -> (8.7595, -88.1894)
  line L2520 (8.7511, -88.1552) -> (8.7542, -88.1723)
  line L2521 (8.75, -88.1381) -> (8.7511, -88.1552)
  line L2522 (8.75, -87.9646) -> (8.75, -88.1381)
  line L2523 (8.7669, -88.2063) -> (8.7764, -88.2232)
  line L2524 (8.8018, -88.2564) -> (8.8176, -88.2727)
  line L2525 (8.8176, -88.2727) -> (8.8355, -88.2888)
  line L2526 (8.8355, -88.2888) -> (8.8556, -88.3046)
  line L2527 (8.8556, -88.3046) -> (8.8777, -88.3202)
  line L2528 (8.8777, -88.3202) -> (8.9019, -88.3354)
  line L2529 (8.9019, -88.3354) -> (8.9282, -88.3503)
  line L2530 (8.9282, -88.3503) -> (8.9566, -88.3648)
  line L2531 (8.9566, -88.3648) -> (8.9871, -88.3789)
  line L2532 (8.9871, -88.3789) -> (9.0196, -88.3925)
  line L2533 (8.8355, -85.1472) -> (8.8556, -85.163)
  line L2534 (8.8556, -85.163) -> (8.8777, -85.1786)
  line L2535 (8.8777, -85.1786) -> (8.9019, -85.1938)
  line L2536 (9.0196, -85.251) -> (9.0542, -85.2642)
  line L2537 (8.9566, -85.2232) -> (8.9871, -85.2373)
  line L2538 (9.0196, -82.1094) -> (9.0542, -82.1226)
  line L2539 (8.9871, -82.0957) -> (9.0196, -82.1094)
  line L2540 (8.9566, -82.0816) -> (8.9871, -82.0957)
  line L2541 (8.9282, -82.0671) -> (8.9566, -82.0816)
  line L2542 (8.9019, -82.0522) -> (8.9282, -82.0671)
  line L2543 (8.8777, -82.037) -> (8.9019, -82.0522)
  line L2544 (8.8556, -82.0215) -> (8.8777, -82.037)
  line L2545 (8.8355, -82.0056) -> (8.8556, -82.0215)
  line L2546 (8.8176, -81.9895) -> (8.8355, -82.0056)
  line L2547 (8.8018, -81.9732) -> (8.8176, -81.9895)
  line L2548 (8.788, -81.9567) -> (8.8018, -81.9732)
  line L2549 (8.7764, -81.94) -> (8.788, -81.9567)
  line L2550 (8.7669, -81.9231) -> (8.7764, -81.94)
  line L2551 (8.7595, -81.9062) -> (8.7669, -81.9231)
  line L2552 (8.7595, -81.4566) -> (8.7669, -81.4397)
  line L2553 (8.7669, -81.4397) -> (8.7764, -81.4228)
  line L2554 (8.7764, -81.4228) -> (8.788, -81.4061)
  line L2555 (8.788, -81.4061) -> (8.8018, -81.3896)
  line L2556 (8.8018, -81.3896) -> (8.8176, -81.3733)
  line L2557 (8.8176, -81.3733) -> (8.8355, -81.3572)
  line L2558 (8.8355, -81.3572) -> (8.8556, -81.3414)
  line L2559 (8.8777, -81.3258) -> (8.9019, -81.3106)
  line L2560 (8.9019, -81.3106) -> (8.9282, -81.2957)
  line L2561 (8.8556, -81.3414) -> (8.8777, -81.3258)
  line L2562 (8.7764, -100.2724) -> (8.788, -100.2557)
  line L2563 (8.788, -100.2557) -> (8.8018, -100.2392)
  line L2564 (8.8018, -100.2392) -> (8.8176, -100.2228)
  line L2565 (8.8176, -100.2228) -> (8.8355, -100.2068)
  line L2566 (8.8355, -100.2068) -> (8.8556, -100.1909)
  line L2567 (8.8556, -100.1909) -> (8.8777, -100.1754)
  line L2568 (8.9019, -100.1602) -> (8.9282, -100.1453)
  line L2569 (8.7669, -100.2892) -> (8.7764, -100.2724)
  line L2570 (8.7595, -100.3062) -> (8.7669, -100.2892)
  line L2571 (8.7542, -100.3232) -> (8.7595, -100.3062)
  line L2572 (8.7511, -100.3403) -> (8.7542, -100.3232)
  line L2573 (8.75, -100.3575) -> (8.7511, -100.3403)
  line L2574 (8.75, -100.531) -> (8.75, -100.3575)
  line L2575 (8.75, -109.281) -> (8.75, -100.531)
  line L2576 (11, -99.3816) -> (11, -98.9602)
  line L2577 (9.0542, -100.0898) -> (11, -99.3816)
  line L2578 (8.9282, -100.1453) -> (8.9566, -100.1308)
  line L2579 (8.9566, -100.1308) -> (8.9871, -100.1167)
  line L2580 (8.9871, -100.1167) -> (9.0196, -100.103)
  line L2581 (9.0196, -100.103) -> (9.0542, -100.0898)
  line L2582 (8.8777, -100.1754) -> (8.9019, -100.1602)
  line L2583 (8.75, -109.281) -> (-1.25, -109.281)
  line L2584 (8.75, -109.281) -> (18.75, -109.281) construction
  line L2585 (-1.25, -109.281) -> (-1.25, 10.75)
  point P0 (0, 0)
  point P1 (8.75, -104.3979)
  point P2 (8.75, -100.4442)
  dimension "d0" = 10
  dimension "d1" = 10
  dimension "d4" = 3.9536
  dimension "d5" = 10
  dimension "d6" = 180
  constraints: 5172 end point, 1887 symmetric about line, 7 horizontal, 3 parallel, 2 collinear, 1 midpoint, 1 perpendicular, 1 point on line, 1 vertical
  measures "d0" distance of L1286.end L1288.start
  measures "d1" distance of L1295.start L1286.end
  measures "d4" distance of point (8.75, -104.398) point (8.75, -100.444)
  measures "d5" distance of L2575.start L2583.end
  measures "d6" angle of L2583 L2584
extrude "押し出し1" add sketch "スケッチ1" along normal blind 10 contours L2018 L2019 L2020 L2021 L2022 L2023 L2024 L2025 L1914 L1913 L1912 L1911 L1910 L1909 L1908 L1907 L1906 L1905 L2026 L2027 L2031 L2032 L2030 L2029 L2028 L1932 L1931 L1930 L1929 L1928 L1927 L1921 L1920 L1926 L1933 L1925 L1924 L1923 L1922 L1915 L1916 L1917 L1918 L1919 L1964 L1965 L1966 L1967 L1970 L1968 L1969 L1957 L1958 L1959 L1960 L1961 L1956 L1962 L1955 L1963 L1954 L1953 L1952 L1951 L1950 L1937 L1936 L1935 L1949 L1948 L1947 L1946 L1945 L1944 L1943 L1942 L1941 L1940 L1939 L1938 L2097 L2098 L2099 L2100 L2101 L2102 L2103 L2104 L2009 L2010 L2011 L2012 L2013 L2014 L2015 L2016 L2017 L2034 L2035 L2037 L2036 L2033 L2008 L2007 L2006 L2005 L2004 L2003 L2001 L2000 L1999 L1998 L2002 L1997 L1996 L1995 L1994 L1993 L1992 L1991 L1990 L1989 L1988 L1987 L1986 L1985 L1984 L1975 L1976 L1977 L1978 L1979 L1980 L1981 L1982 L1983 L1974 L1973 L1972 L1971 L1428 L1427 L1422 L1421 L1420 L1419 L1426 L1425 L1424 L1423 L1408 L1409 L1410 L1411 L1412 L1413 L1414 L1415 L1416 L1417 L1808 L1807 L1809 L1806 L1805 L1804 L1803 L1801 L1800 L1799 L1798 L1802 L1797 L1796 L1795 L1780 L1781 L1782 L1784 L1786 L1785 L1783 L1794 L1793 L1792 L1791 L1790 L1789 L1788 L1787 L1771 L1772 L1773 L1774 L1775 L1779 L1817 L1816 L1815 L1814 L1813 L1776 L1777 L1778 L1769 L1768 L1767 L1766 L1765 L1770 L1764 L1757 L1758 L1759 L1760 L1761 L1763 L1762 L1749 L1754 L1755 L1756 L1753 L1752 L1751 L1750 L1748 L1747 L1746 L1745 L1744 L1743 L1742 L1741 L1740 L1739 L1738 L1737 L1736 L1735 L1592 L1591 L1589 L1588 L1587 L1586 L1585 L1584 L1583 L1582 L1581 L1580 L1579 L1578 L1577 L1576 L1575 L1574 L1573 L1572 L1571 L1570 L1566 L1567 L1569 L1564 L1563 L1562 L1561 L1560 L1565 L1559 L1558 L1557 L1732 L1734 L1568 L1812 L1811 L1810 L1590 L1556 L1555 L1554 L1553 L1552 L1551 L1550 L1549 L1547 L1546 L1545 L1544 L1543 L1548 L1542 L1541 L1540 L1539 L1538 L1537 L1536 L1528 L1527 L1529 L1530 L1531 L1532 L1535 L1533 L1534 L1526 L1525 L1524 L1523 L1522 L1521 L1520 L1519 L1429 L1720 L1719 L1889 L1888 L1887 L1886 L1904 L1903 L1902 L1901 L1900 L1899 L1898 L1897 L1896 L1895 L1894 L1893 L1890 L1891 L1892 L1885 L1875 L1876 L1877 L1878 L1879 L1880 L1881 L1882 L1883 L1884 L1870 L1869 L1871 L1872 L1873 L1874 L1718 L1721 L1717 L1716 L1857 L1858 L1859 L1860 L1861 L1862 L1863 L1864 L1865 L1866 L1867 L1868 L2084 L2085 L2086 L2094 L2087 L2093 L2092 L2091 L2095 L2090 L2089 L2088 L1856 L1848 L1851 L1850 L1849 L1852 L1853 L1854 L1838 L1839 L1840 L1841 L1847 L1842 L1843 L1844 L1845 L1846 L1855 L1837 L1836 L1835 L1834 L1833 L1832 L1831 L2060 L2061 L2062 L2063 L2064 L2065 L2066 L2068 L2067 L2059 L2082 L2083 L2081 L2080 L2079 L2078 L2049 L2050 L2051 L2052 L2053 L2054 L2055 L2056 L2057 L2058 L2048 L2047 L2045 L2044 L2038 L2046 L2043 L2042 L2041 L2040 L2039 L2069 L2070 L2071 L2072 L2073 L2074 L2075 L2076 L2077 L2105 L2106 L2107 L2108 L2109 L2110 L2111 L2112 L2113 L2114 L2115 L1828 L1827 L1826 L1829 L1825 L1824 L1823 L1822 L1821 L1820 L1830 L1715 L1714 L1713 L1712 L1819 L1818 L1711 L1710 L1709 L1708 L1707 L1706 L1705 L1704 L1703 L1702 L1700 L1701 L1693 L1699 L1698 L1697 L1696 L1695 L1694 L1682 L1683 L1684 L1692 L1685 L1686 L1687 L1681 L1678 L1679 L1680 L1436 L1437 L1438 L1439 L1440 L1441 L1442 L1443 L1688 L1689 L1690 L1691 L1669 L1670 L1671 L1672 L1673 L1674 L1675 L1677 L1657 L1676 L1647 L1651 L1650 L1649 L1648 L1658 L1659 L1660 L1668 L1646 L1661 L1662 L1663 L1664 L1665 L1666 L1656 L1655 L1654 L1653 L1635 L1634 L1633 L1632 L1652 L1667 L1631 L1630 L1629 L1620 L1621 L1622 L1623 L1624 L1618 L1619 L1625 L1628 L1626 L1627 L1642 L1644 L1645 L1643 L1640 L1639 L1638 L1637 L1636 L1641 L1617 L1616 L1615 L1614 L1613 L1612 L1611 L1610 L1609 L1608 L1607 L1606 L1601 L1602 L1603 L1604 L1605 L1600 L1599 L1598 L1722 L1723 L1731 L1724 L1725 L1726 L1727 L1728 L1729 L1730 L1595 L1596 L1597 L1594 L1593 L1518 L1517 L1516 L1515 L1514 L1513 L1512 L1511 L1510 L1509 L1508 L1507 L1506 L1444 L1505 L1445 L1504 L1499 L1500 L1501 L1502 L1487 L1503 L1488 L1489 L1490 L1491 L1492 L1493 L1494 L1482 L1495 L1496 L1498 L1497 L1486 L1485 L1484 L1483 L1474 L1473 L1475 L1476 L1477 L1478 L1479 L1481 L1480 L1471 L1470 L1472 L1469 L1468 L1467 L1466 L1465 L1464 L1463 L1462 L1461 L1460 L1459 L1458 L1446 L1456 L1455 L1454 L1453 L1452 L1451 L1450 L1449 L1448 L1447 L1457 L1430 L1431 L1433 L1434 L1432 L1435 L1309 L1308 L1307 L1306 L1305 L1304 L1303 L1302 L1301 L1300 L1299 L1298 L1297 L1296 L1318 L1317 L1316 L1315 L1319 L1314 L1313 L1312 L1311 L1310 L1328 L1327 L1326 L1329 L1325 L1324 L1323 L1322 L1321 L1320 L1337 L1338 L1341 L1342 L1343 L1340 L1339 L1336 L1335 L1334 L1332 L1333 L1331 L1330 L1344 L1345 L1346 L1347 L1348 L1349 L1350 L1351 L1352 L1357 L1353 L1354 L1355 L1356 L1368 L1367 L1366 L1365 L1364 L1363 L1362 L1361 L1360 L1359 L1358 L1407 L1402 L1404 L1405 L1406 L1401 L1403 L1400 L1399 L1398 L1397 L1373 L1374 L1375 L1376 L1377 L1378 L1379 L1384 L1380 L1381 L1382 L1383 L2279 L2278 L2277 L2276 L2275 L2274 L1369 L1372 L1370 L1371 L2273 L2272 L2271 L2270 L2269 L2268 L2267 L2266 L2230 L2232 L2229 L2231 L2227 L2226 L2225 L2228 L2224 L2223 L2222 L2221 L2220 L2219 L2218 L2217 L2216 L2215 L2214 L2213 L2212 L2211 L1385 L1386 L2209 L2210 L2208 L2207 L2206 L2205 L2204 L2203 L2202 L2201 L2200 L2199 L2198 L2197 L2196 L2195 L2194 L2193 L2192 L2191 L2185 L2186 L2187 L2188 L2190 L2189 L2184 L2183 L2182 L2181 L2180 L2179 L1393 L1387 L1388 L1389 L1390 L1391 L2161 L2160 L2159 L2158 L2157 L2170 L2243 L2242 L2241 L2240 L2239 L2238 L2244 L2237 L2236 L2235 L2234 L2233 L2174 L2177 L2178 L2176 L2175 L2171 L2172 L2173 L2169 L2168 L2167 L2166 L2165 L2164 L2163 L2162 L2156 L2155 L2154 L2153 L2152 L2151 L2150 L2149 L2148 L2147 L2146 L2145 L2135 L2134 L2133 L2132 L2131 L2130 L2129 L2128 L2127 L2126 L2125 L2124 L2245 L2246 L2247 L2248 L2249 L2144 L2143 L2142 L2141 L2140 L2139 L2138 L2136 L2137 L2116 L2117 L2118 L2119 L2120 L2121 L2122 L2123 L2250 L2251 L2252 L2253 L2254 L2255 L2256 L2257 L2259 L2258 L2260 L2265 L2261 L2262 L2263 L2264 L2406 L2407 L2408 L2409 L2410 L2411 L2412 L2421 L2420 L2419 L2418 L2417 L2416 L2415 L2414 L2413 L2436 L2435 L2434 L2433 L2432 L2422 L2431 L2430 L2429 L2437 L2428 L2427 L2426 L2425 L2424 L2423 L2447 L2446 L2445 L2444 L2443 L2442 L2441 L2440 L2439 L2438 L2449 L2454 L2455 L2453 L2448 L2452 L2451 L2450 L2560 L2559 L2561 L2558 L2557 L2556 L2555 L2554 L2553 L2552 L2463 L2462 L2461 L2460 L2459 L2458 L2457 L2456 L2551 L2550 L2549 L2548 L2547 L2546 L2545 L2544 L2543 L2542 L2541 L2540 L2539 L2538 L2465 L2466 L2467 L2464 L2481 L2480 L2479 L2478 L2477 L2476 L2475 L2474 L2473 L2472 L2471 L2470 L2469 L2468 L2482 L2483 L2484 L2485 L2486 L2487 L2488 L2489 L2495 L2492 L2493 L2491 L2490 L2494 L2533 L2534 L2535 L2496 L2497 L2537 L2405 L2536 L2401 L2403 L2404 L2402 L2501 L2500 L2499 L2502 L2503 L2504 L2510 L2505 L2506 L2507 L2508 L2509 L2498 L2514 L2513 L2512 L2511 L2515 L2522 L2521 L2520 L2519 L2518 L2523 L2517 L2516 L2524 L2525 L2526 L2527 L2528 L2529 L2530 L2531 L2532 L2280 L2281 L2287 L2286 L2285 L2284 L2283 L2282 L2288 L2290 L2291 L2292 L2293 L2294 L2295 L2296 L2299 L2289 L1394 L1396 L1395 L2324 L2297 L2298 L2300 L2301 L2302 L2303 L2304 L2305 L2306 L2307 L2308 L2309 L2310 L2311 L2312 L2313 L2314 L2315 L2316 L2322 L2321 L2320 L2319 L2318 L2317 L2323 L2331 L2332 L2333 L2334 L2335 L2336 L2337 L2338 L2339 L2325 L2330 L2340 L2326 L2327 L2329 L2341 L2342 L2343 L2346 L2344 L2345 L2370 L2371 L2372 L2373 L2374 L2369 L2366 L2367 L2368 L2391 L2392 L2393 L2394 L2395 L2399 L2398 L2397 L2396 L2400 L2347 L2348 L2349 L2350 L2358 L2351 L2352 L2353 L2354 L2375 L2355 L2356 L2357 L2365 L2359 L2360 L2361 L2362 L2363 L2364 L2376 L2382 L2377 L2378 L2379 L2380 L2381 L2383 L2384 L2390 L2385 L2386 L2387 L2388 L2389 L2576 L2577 L2581 L2580 L2579 L2578 L2568 L2582 L2567 L2566 L2565 L2564 L2563 L2562 L2569 L2570 L2571 L2572 L2573 L2574 L2575 L2583 L2585 L1295 L1286 L1287 L1288 L767 L768 L779 L778 L777 L766 L775 L776 L774 L773 L772 L771 L770 L769 L762 L763 L764 L765 L761 L760 L757 L759 L758 L746 L745 L744 L743 L742 L739 L738 L737 L736 L735 L741 L740 L756 L755 L749 L748 L747 L754 L753 L752 L751 L750 L726 L727 L728 L729 L730 L731 L732 L733 L734 L725 L722 L721 L723 L720 L724 L719 L718 L717 L716 L715 L702 L701 L700 L707 L713 L712 L714 L711 L710 L709 L708 L706 L705 L704 L703 L691 L692 L693 L699 L694 L695 L696 L697 L698 L682 L689 L683 L681 L684 L685 L686 L687 L688 L679 L678 L677 L676 L675 L674 L673 L672 L671 L670 L669 L668 L667 L666 L680 L786 L785 L784 L783 L782 L781 L780 L787 L665 L664 L663 L662 L661 L660 L659 L658 L657 L656 L650 L651 L652 L653 L654 L655 L649 L648 L647 L646 L645 L644 L1127 L1126 L1125 L1136 L1135 L1134 L1133 L1132 L1131 L1130 L1129 L1128 L1147 L1139 L1140 L1138 L1137 L1141 L1142 L1143 L1144 L1145 L1146 L1162 L1163 L1161 L1160 L1159 L1158 L1157 L1156 L1155 L1148 L1149 L1150 L1152 L1154 L1153 L1151 L1285 L1284 L1283 L1282 L1281 L1280 L1279 L1278 L1277 L1164 L1165 L1166 L1167 L1168 L1172 L1169 L1170 L1171 L1173 L1174 L1175 L1176 L1177 L1178 L1179 L1180 L1181 L1187 L1182 L1183 L1184 L1185 L1186 L1194 L1188 L1189 L1190 L1191 L1192 L1193 L1199 L1198 L1200 L1197 L1196 L1195 L1212 L1211 L1210 L1209 L1208 L1207 L1206 L1205 L1204 L1203 L1202 L1201 L1215 L1216 L1217 L1218 L1226 L1222 L1223 L1224 L1225 L1221 L1220 L1219 L1213 L1214 L1229 L1230 L1228 L1227 L1236 L1235 L1234 L1233 L1232 L1231 L1237 L1245 L1244 L1243 L1242 L1241 L1240 L1239 L1246 L1238 L1251 L1250 L1252 L1249 L1248 L1247 L1260 L1259 L1258 L1257 L1256 L1255 L1254 L1253 L1268 L1269 L1270 L1271 L1272 L1273 L1274 L1275 L1276 L1267 L1266 L1265 L1264 L1263 L1262 L1261 L821 L820 L819 L818 L817 L812 L811 L816 L822 L815 L814 L813 L810 L809 L808 L807 L806 L798 L805 L804 L803 L802 L801 L800 L799 L788 L789 L790 L791 L792 L796 L793 L794 L795 L823 L824 L825 L826 L827 L828 L838 L837 L836 L835 L834 L833 L832 L831 L830 L829 L839 L840 L841 L842 L843 L844 L845 L846 L847 L848 L849 L850 L851 L852 L853 L854 L855 L856 L857 L858 L859 L860 L866 L861 L862 L863 L864 L865 L964 L963 L962 L961 L960 L959 L958 L957 L867 L868 L869 L870 L871 L872 L873 L874 L875 L876 L877 L878 L882 L879 L880 L881 L883 L884 L885 L886 L887 L888 L889 L890 L891 L892 L893 L894 L895 L896 L897 L898 L903 L904 L902 L901 L900 L899 L907 L908 L909 L910 L916 L911 L912 L913 L914 L915 L906 L905 L925 L924 L917 L923 L922 L921 L920 L919 L918 L926 L927 L928 L929 L930 L934 L931 L932 L933 L938 L935 L936 L937 L946 L945 L944 L943 L942 L941 L940 L939 L955 L954 L956 L953 L952 L951 L950 L949 L948 L947 L1007 L1006 L1005 L1004 L1003 L1002 L1001 L1000 L999 L998 L997 L996 L1008 L1009 L1010 L1011 L1013 L1012 L1124 L1123 L1122 L1121 L1025 L1024 L1023 L1022 L1021 L1020 L1019 L1018 L1017 L1016 L1015 L1014 L1026 L1027 L1028 L1029 L1030 L1031 L1032 L1033 L1034 L1035 L1036 L1037 L1038 L1039 L1040 L1041 L1043 L1042 L1044 L1045 L1046 L1047 L1048 L1049 L1050 L1051 L1053 L1052 L1063 L1062 L1061 L1060 L1059 L1058 L1057 L1056 L1055 L1054 L1071 L1070 L1069 L1068 L1067 L1066 L1065 L1064 L1079 L1080 L1081 L1082 L1076 L1077 L1078 L1083 L1084 L1087 L1085 L1086 L1072 L1073 L1074 L1075 L1088 L1089 L1090 L1091 L1093 L1092 L1099 L1098 L1097 L1096 L1095 L1094 L995 L994 L993 L992 L991 L990 L989 L988 L987 L986 L985 L984 L983 L979 L980 L981 L982 L978 L977 L975 L976 L1106 L1105 L1120 L1104 L1103 L1107 L1102 L1101 L1100 L966 L967 L968 L969 L970 L971 L972 L973 L965 L974 L1115 L1116 L1117 L1118 L1119 L1114 L1113 L1112 L1111 L1110 L1109 L1108 L324 L325 L326 L327 L328 L329 L332 L355 L350 L349 L348 L347 L346 L330 L331 L333 L344 L345 L351 L354 L353 L352 L399 L398 L397 L396 L395 L394 L393 L392 L343 L335 L334 L336 L337 L338 L339 L340 L341 L342 L356 L357 L358 L359 L360 L361 L362 L363 L364 L391 L383 L384 L385 L386 L387 L388 L382 L389 L381 L390 L380 L379 L378 L377 L368 L367 L366 L365 L375 L376 L374 L373 L372 L371 L370 L369 L468 L458 L457 L456 L459 L460 L461 L462 L463 L464 L465 L466 L467 L470 L471 L472 L469 L473 L474 L475 L476 L477 L482 L481 L480 L479 L478 L483 L438 L437 L436 L435 L434 L433 L432 L439 L431 L429 L428 L427 L426 L430 L425 L424 L406 L405 L404 L403 L402 L401 L400 L407 L415 L423 L416 L417 L418 L419 L420 L421 L422 L414 L413 L412 L411 L410 L409 L408 L441 L440 L446 L447 L448 L449 L454 L453 L452 L451 L455 L450 L445 L444 L443 L442 L564 L565 L566 L567 L568 L569 L570 L571 L572 L573 L574 L643 L638 L639 L640 L633 L634 L635 L637 L641 L642 L636 L592 L593 L594 L595 L596 L597 L598 L603 L602 L601 L600 L599 L604 L591 L590 L575 L576 L577 L578 L579 L580 L581 L582 L583 L584 L585 L586 L587 L588 L589 L615 L616 L617 L618 L620 L619 L605 L613 L614 L612 L611 L610 L609 L608 L607 L606 L562 L561 L560 L559 L558 L557 L563 L556 L539 L538 L537 L536 L535 L534 L533 L532 L531 L530 L529 L528 L527 L523 L524 L525 L522 L526 L625 L626 L627 L628 L631 L630 L629 L624 L632 L623 L622 L621 L520 L521 L519 L518 L517 L516 L515 L514 L513 L512 L511 L510 L509 L508 L507 L506 L505 L504 L503 L502 L492 L493 L494 L495 L496 L497 L498 L499 L500 L501 L491 L490 L489 L488 L487 L486 L541 L540 L554 L553 L552 L555 L551 L550 L549 L548 L547 L546 L545 L544 L543 L542 L484 L485 L167 L168 L169 L170 L181 L180 L179 L178 L177 L171 L172 L176 L175 L174 L173 L182 L163 L164 L165 L166 L183 L184 L185 L186 L187 L188 L189 L193 L194 L195 L192 L191 L190 L196 L197 L198 L199 L200 L201 L202 L242 L241 L240 L239 L238 L237 L203 L204 L205 L211 L206 L207 L208 L209 L210 L236 L233 L234 L232 L235 L231 L230 L229 L228 L227 L226 L213 L212 L218 L219 L220 L221 L224 L225 L223 L222 L217 L216 L215 L214 L285 L286 L287 L288 L289 L296 L290 L291 L292 L293 L294 L295 L297 L298 L299 L300 L301 L302 L318 L319 L321 L322 L320 L274 L273 L272 L271 L270 L269 L284 L283 L282 L281 L280 L279 L278 L277 L276 L275 L254 L253 L252 L251 L250 L255 L268 L267 L266 L265 L264 L263 L262 L261 L260 L259 L258 L257 L256 L246 L248 L249 L247 L245 L244 L243 L303 L304 L305 L317 L306 L307 L308 L309 L310 L311 L312 L313 L314 L315 L316 L122 L123 L124 L125 L135 L134 L133 L132 L131 L130 L129 L128 L127 L126 L82 L83 L84 L85 L86 L87 L88 L89 L90 L91 L92 L93 L94 L95 L98 L99 L100 L97 L96 L101 L102 L103 L104 L105 L106 L107 L108 L109 L110 L111 L112 L113 L114 L121 L115 L116 L117 L118 L119 L120 L161 L158 L157 L159 L156 L160 L155 L154 L153 L152 L151 L150 L137 L136 L142 L143 L144 L145 L146 L147 L148 L149 L141 L140 L139 L138 L50 L51 L52 L53 L61 L60 L59 L58 L57 L56 L55 L54 L41 L42 L43 L44 L45 L46 L47 L48 L71 L49 L72 L62 L63 L64 L65 L66 L67 L68 L69 L70 L73 L74 L80 L75 L76 L77 L78 L79 L32 L33 L34 L38 L37 L36 L35 L20 L21 L22 L23 L24 L39 L25 L26 L27 L28 L29 L30 L31 L19 L18 L17 L16 L15 L14 L13 L12 L11 L10 L9 L8 L7 L6 L5 L4 L3 L2 L1 L0
sketch "スケッチ14" plane through (0, 0, 10) normal (0, 0, 1) x (1, 0, 0)
  line L0 (-1.25, 109.281) -> (-1.25, -109.281) projected
  line L1 (-1.25, -109.281) -> (8.75, -109.281) projected
  line L2 (-1.25, 109.281) -> (-0.25, 109.281)
  line L3 (-0.25, 109.281) -> (-0.25, -109.281)
  line L4 (-0.25, -109.281) -> (-1.25, -109.281)
  line L5 (-1.25, -109.281) -> (-1.25, 109.281)
  point P0 (0, 0)
  dimension "d69" = 1
  constraints: 8 end point, 2 parallel, 1 horizontal, 1 perpendicular, 1 point on line
  measures "d69" distance of L3.end L4.end
extrude "押し出し12" cut sketch "スケッチ14" against normal blind 10
sketch "スケッチ15" plane through (0, 0, 10) normal (0, 0, 1) x (1, 0, 0)
  line L0 (-0.25, 109.281) -> (-0.25, -109.281) projected
  line L1 (-0.25, 109.281) -> (8.75, 109.281)
  line L2 (8.75, 109.281) -> (8.75, 101.281)
  line L3 (8.75, 101.281) -> (-0.25, 101.281)
  line L4 (-0.25, 101.281) -> (-0.25, 109.281)
  line L5 (-0.25, -109.281) -> (8.75, -109.281) projected
  line L6 (8.75, -109.281) -> (-0.25, -109.281)
  line L7 (-0.25, -109.281) -> (-0.25, -101.281)
  line L8 (-0.25, -101.281) -> (8.75, -101.281)
  line L9 (8.75, -101.281) -> (8.75, -109.281)
  point P0 (0, 0)
  point P1 (-0.25, 101.281)
  dimension "d72" = 9
  dimension "d73" = 8
  dimension "d74" = 9
  dimension "d75" = 8
  constraints: 16 end point, 4 parallel, 2 horizontal, 2 perpendicular
  measures "d72" distance of L2.end L3.end
  measures "d73" distance of L1.end L2.end
  measures "d74" distance of L7.end L8.end
  measures "d75" distance of L6.end L7.end
extrude "押し出し13" cut sketch "スケッチ15" against normal blind 10